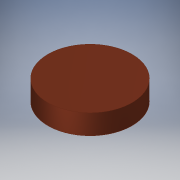
# Autodesk Inventor part: plug
Saved by Autodesk Inventor 2018 (Build 220112000, 112)
## iProperties
Created: 2019-03-06
Part Number: plug
Material: Copper
Document SubType Name: Modeling
Designer: Admin
Density: 8.94 g/cm^3
Appearance: Copper - Satin
Author: Admin
Autodesk Inventor part; units mm, degrees
ref_plane "YZ Plane" through (0, 0, 0) normal (1, 0, 0) x (0, 1, 0)
ref_plane "XZ Plane" through (0, 0, 0) normal (0, 1, 0) x (-1, 0, 0)
ref_plane "XY Plane" through (0, 0, 0) normal (0, 0, 1) x (1, 0, 0)
sketch "Sketch1" plane through (0, 0, 0) normal (0, 1, 0) x (-1, 0, 0)
  circle A0 centre (0, 0) radius 13.335
  dimension "d0" = 26.67
  constraints: 1 centre point, 1 coincident
  measures "d0" diameter of A0
extrude "Extrusion1" add sketch "Sketch1" along normal blind 6.35
body "Solid1"
